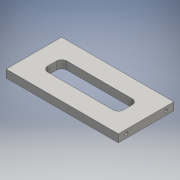
# Autodesk Inventor part: body2
Saved by Autodesk Inventor 2016 SP1 (Build 200210100, 210)
## iProperties
Created: 2018-04-30
Part Number: body2
Material: 一般
Document SubType Name: Modeling
Designer: kobay
Density: 1 g/cm^3
Appearance: 既定
Author: kobay
Autodesk Inventor part; units mm, degrees
ref_plane "YZ Plane" through (0, 0, 0) normal (1, 0, 0) x (0, 1, 0)
ref_plane "XZ Plane" through (0, 0, 0) normal (0, 1, 0) x (-1, 0, 0)
ref_plane "XY Plane" through (0, 0, 0) normal (0, 0, 1) x (1, 0, 0)
sketch "スケッチ1" plane through (0, 0, 0) normal (0, 0, 1) x (1, 0, 0)
  line L0 (0, 0) -> (85, 0)
  line L1 (85, 0) -> (85, 42)
  line L2 (85, 42) -> (0, 42)
  line L3 (0, 42) -> (0, 0)
  dimension "d0" = 85
  dimension "d1" = 42
  constraints: 8 end point, 2 parallel, 1 horizontal, 1 perpendicular
  measures "d0" distance of L2.end L1.end
  measures "d1" distance of L1.end L0.end
extrude "押し出し1" add sketch "スケッチ1" along normal blind 6
sketch "スケッチ2" plane through (0, 0, 0) normal (-1, 0, 0) x (0, 0, 1)
  circle A0 centre (3, 36) radius 1.2
  circle A1 centre (3, 6) radius 1.2
  line L0 (0, 42) -> (6, 42) projected
  line L1 (0, 0) -> (6, 0) projected
  dimension "d4" = 2.4
  dimension "d5" = 2.4
  dimension "d6" = 6
  dimension "d7" = 6
  constraints: 2 centre point
  measures "d4" diameter of A0
  measures "d5" diameter of A1
  measures "d6" distance from line of A0.centre L0
  measures "d7" distance from line of L1 A1.centre
extrude "押し出し2" cut sketch "スケッチ2" against normal blind 8
sketch "スケッチ3" plane through (85, 0, 0) normal (1, 0, 0) x (0, 0, -1)
  circle A0 centre (-3, 6) radius 1.2 projected
  circle A1 centre (-3, 6) radius 1.2
  circle A2 centre (-3, 36) radius 1.2 projected
  circle A3 centre (-3, 36) radius 1.2
  point P0 (0, 0)
  constraints: 2 centre point, 2 coincident
extrude "押し出し3" cut sketch "スケッチ3" against normal blind 8
sketch "スケッチ4" plane through (0, 0, 6) normal (0, 0, 1) x (1, 0, 0)
  line L0 (0, 0) -> (85, 0) projected
  line L1 (85, 0) -> (85, 42) projected
  line L2 (85, 42) -> (0, 42) projected
  line L3 (0, 42) -> (0, 0) projected
  line L4 (13.6951, 28.3049) -> (71.3049, 28.3049)
  line L5 (71.3049, 28.3049) -> (71.3049, 13.6951)
  line L6 (71.3049, 13.6951) -> (13.6951, 13.6951)
  line L7 (13.6951, 13.6951) -> (13.6951, 28.3049)
  constraints: 8 end point, 3 other
extrude "押し出し4" cut sketch "スケッチ4" against normal blind 10 contours L4 L5 L6 L7
fillet "フィレット1" radius 4 4 edges at (13.6951, 28.3049, 3) (13.6951, 13.6951, 3) (71.3049, 13.6951, 3) (71.3049, 28.3049, 3)
